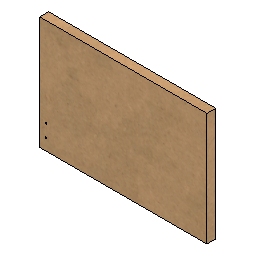
XAxisDriveBase (Autodesk Fusion 360 design; units mm, degrees)
Autodesk Fusion 360 part; units mm, degrees
sketch "Sketch1" plane through (-32.5, 282.8925, 28) normal (0, 0, 1) x (0, 1, 0)
  line L0 (-232.4915, -49) -> (-232.4915, -16)
  line L1 (-232.4915, -16) -> (-271.8915, -16)
  line L2 (-271.8915, -16) -> (-271.8915, -49)
  line L3 (-271.8915, -49) -> (-232.4915, -49)
  circle A0 centre (-239.1915, -45.5) radius 1.65
  circle A1 centre (-265.1915, -45.5) radius 1.65
  circle A2 centre (-239.1915, -19.5) radius 1.65
  circle A3 centre (-265.1915, -19.5) radius 1.65
  line L4 (-286.4915, 275) -> (-56.4915, 275)
  line L5 (-56.4915, 275) -> (-56.4915, -65)
  line L6 (-56.4915, -65) -> (-286.4915, -65)
  line L7 (-286.4915, -65) -> (-286.4915, 275)
  line L8 (-271.8915, 49) -> (-271.8915, 16) construction
  line L9 (-71.0915, 16) -> (-71.0915, 49) construction
  line L10 (-271.8915, 49) -> (-71.0915, 49) construction
  line L11 (-71.0915, 49) -> (-71.0915, 16) construction
  line L12 (-71.0915, 16) -> (-271.8915, 16) construction
  line L13 (-271.8915, 16) -> (-271.8915, 49) construction
  line L14 (-171.4915, 49) -> (-171.4915, 16) construction
  line L15 (-357.8915, -65) -> (792.1085, -65) construction
  dimension "d86" = 115
  dimension "d87" = 115
  dimension "d88" = 340
  constraint horizontal L4
  constraint vertical L5
  constraint horizontal L6
  constraint vertical L7
  constraint horizontal L10
  constraint vertical L11
  constraint horizontal L12
  constraint vertical L13
  constraint coincident L9.start L11.end
  constraint coincident L8.start L10.start
  constraint midpoint L10 L14.start
  constraint midpoint L12 L14.end
  constraint collinear L6 L15
  measures "d86" distance of L5 L14
  measures "d87" distance of L7 L14
  measures "d88" distance of L4.end L5.end
extrude "Extrude1" add sketch "Sketch1" along normal blind 18 contours L0 L1 L2 L3 | A0 | A1 | A2 | A3 | L4 L5 L6 L7
sketch "Sketch2" plane through (-145.436, 0, 46) normal (0, 0, 1) x (1, 0, 0)
  line L0 (-358.164, -65) -> (-128.164, -65)
  line L1 (-128.164, -65) -> (-128.164, 275)
  line L2 (-128.164, 275) -> (-358.164, 275)
  line L3 (-358.164, 275) -> (-358.164, -65)
  circle A0 centre (-310.864, 45.5) radius 1.65
  circle A1 centre (-336.864, 45.5) radius 1.65
  circle A2 centre (-336.864, 19.5) radius 1.65
  circle A3 centre (-310.864, 19.5) radius 1.65
  circle A4 centre (-336.864, -19.5) radius 1.65
  circle A5 centre (-310.864, -19.5) radius 1.65
  circle A6 centre (-336.864, -45.5) radius 1.65
  circle A7 centre (-310.864, -45.5) radius 1.65
  circle A8 centre (-175.464, 45.5) radius 1.65
  circle A9 centre (-149.464, 45.5) radius 1.65
  circle A10 centre (-175.464, 19.5) radius 1.65
  circle A11 centre (-149.464, 19.5) radius 1.65
  circle A12 centre (-175.464, -19.5) radius 1.65
  circle A13 centre (-149.464, -19.5) radius 1.65
  circle A14 centre (-175.464, -45.5) radius 1.65
  circle A15 centre (-149.464, -45.5) radius 1.65
  point P0 (-336.864, 47.15)
  point P1 (-310.864, 47.15)
extrude "Extrude2" cut sketch "Sketch2" against normal through all contours A0 | A1 | A2 | A3 | A4 | A5 | A6 | A7 | A8 | A9 | A10 | A11 | A12 | A13 | A14 | A15
equation "d89 = BoardThickness"
equation "BoardThickness = 18 mm"
